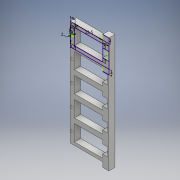
# Autodesk Inventor part: ServoHolder
Saved by Autodesk Inventor 2017 (Build 210142000, 142)
## iProperties
Created: 2017-12-02
Part Number: ServoHolder
Material: Generic
Document SubType Name: Modeling
Designer: Max
Density: 1 g/cm^3
Appearance: Default
Author: Max
Autodesk Inventor part; units mm, degrees
ref_plane "YZ Plane" through (0, 0, 0) normal (1, 0, 0) x (0, 1, 0)
ref_plane "XZ Plane" through (0, 0, 0) normal (0, 1, 0) x (-1, 0, 0)
ref_plane "XY Plane" through (0, 0, 0) normal (0, 0, 1) x (1, 0, 0)
sketch "Sketch1" plane through (0, 0, 0) normal (0, 1, 0) x (-1, 0, 0)
  line L0 (0, 0) -> (27.5, 0)
  line L1 (27.5, 0) -> (27.5, -2.5)
  line L2 (27.5, -2.5) -> (5, -2.5)
  line L3 (5, -2.5) -> (5, -15.5)
  line L4 (5, -15.5) -> (27.5, -15.5)
  line L5 (27.5, -15.5) -> (27.5, -18)
  line L6 (27.5, -18) -> (0, -18)
  line L7 (0, -18) -> (0, 0)
  line L8 (27.5, -2.5) -> (28, -2.5)
  line L9 (28, -2.5) -> (28, -15.5)
  line L10 (28, -15.5) -> (27.5, -15.5)
  line L11 (27.5, 0) -> (31.5, 0)
  line L12 (31.5, 0) -> (31.5, -18)
  line L13 (31.5, -18) -> (27.5, -18)
  circle A0 centre (30, -9) radius 1
  line L14 (5, -5.5) -> (0, -5.5)
  line L15 (5, -12.5) -> (0, -12.5)
  line L16 (0, 0) -> (0, 4)
  line L17 (0, 4) -> (5, 4)
  line L18 (5, 4) -> (5, 0)
  line L19 (0, -18) -> (0, -22)
  line L20 (0, -22) -> (5, -22)
  line L21 (5, -22) -> (5, -18)
  line L22 (0.9553, -12.5) -> (0.9553, -5.5)
  dimension "d1" = 2.5
  dimension "d2" = 22.5
  dimension "d4" = 2.5
  dimension "d5" = 5
  dimension "d9" = 13
  dimension "d16" = 0.5
  dimension "d17" = 4
  dimension "d19" = 2
  dimension "d20" = 6.5
  dimension "d21" = 3
  dimension "d22" = 3
  dimension "d23" = 4
  dimension "d24" = 4
  constraints: 46 end point, 16 perpendicular, 8 point on line, 4 horizontal, 2 parallel, 2 vertical, 1 centre point
  measures "d1" distance of L0.end L1.end
  measures "d2" distance of L1.end L2.end
  measures "d4" distance of L4.end L5.end
  measures "d5" distance between parallel lines of L7 L3
  measures "d9" distance of L4.end L1.end
  measures "d16" distance of L1.end L8.end
  measures "d17" distance of L0.end L11.end
  measures "d19" diameter of A0
  measures "d20" distance from line of L2 A0.centre
  measures "d21" distance from line of L14 L2.end
  measures "d22" distance from line of L3.end L15
  measures "d23" distance of L0.start L16.end
  measures "d24" distance of L6.end L19.end
extrude "Extrusion1" add sketch "Sketch1" along normal blind 5 contours L16 L17 L18 L0 | L0 L1 L2 L3 L14 L7 | L14 L22 L15 L7 | L11 L12 L13 L5 L10 L9 L8 L1 | L15 L3 L4 L5 L6 L7 | L6 L21 L20 L19
pattern_linear "Rectangular Pattern1" count 5 spacing 17 along (0, 0, -1)
body "Solid1"
